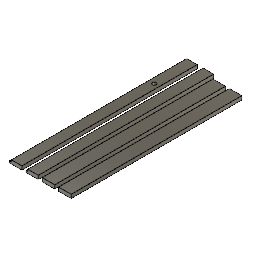
side (Autodesk Fusion 360 design; units mm, degrees)
Autodesk Fusion 360 part; units mm, degrees
sketch "Sketch1" plane through (0, 0, 0) normal (0, 0, 1) x (1, 0, 0)
  line L0 (0, 0) -> (33, 0)
  line L1 (33, 0) -> (33, 460)
  line L2 (33, 460) -> (0, 460)
  line L3 (0, 460) -> (0, 0)
  line L4 (76, 460) -> (43, 460)
  line L5 (43, 460) -> (43, 0)
  line L6 (43, 0) -> (76, 0)
  line L7 (76, 0) -> (76, 460)
  line L8 (86, 0) -> (119, 0)
  line L9 (119, 0) -> (119, 448)
  line L10 (119, 448) -> (86, 448)
  line L11 (86, 448) -> (86, 0)
  line L12 (129, 0) -> (162, 0)
  line L13 (162, 0) -> (162, 448)
  line L14 (162, 448) -> (129, 448)
  line L15 (129, 448) -> (129, 0)
  circle A0 centre (20, 360) radius 5
  line L16 (5, 0) -> (5, 460)
  line L17 (48, 460) -> (48, 0)
  dimension "d1" = 33
  dimension "d2" = 460
  dimension "d3" = 33
  dimension "d4" = 460
  dimension "d5" = 10
  dimension "d6" = 33
  dimension "d8" = 10
  dimension "d9" = 33
  dimension "d10" = 448
  dimension "d11" = 10
  dimension "d14" = 10
  dimension "d15" = 20
  dimension "d16" = 100
  dimension "d19" = 5
  dimension "d20" = 5
  constraint horizontal L0
  constraint vertical L1
  constraint horizontal L2
  constraint vertical L3
  constraint coincident L0.start L3.end
  constraint horizontal L6
  constraint vertical L7
  constraint horizontal L4
  constraint vertical L5
  constraint horizontal L8
  constraint vertical L9
  constraint horizontal L10
  constraint vertical L11
  constraint horizontal L12
  constraint vertical L13
  constraint horizontal L14
  constraint vertical L15
  constraint coincident L0 L16.start
  constraint coincident L2 L16.end
  constraint perpendicular L2 L16
  constraint coincident L4 L17.start
  constraint coincident L6 L17.end
  constraint perpendicular L6 L17
  measures "d1" distance of L0.start L0.end
  measures "d2" distance of L0.start L2.end
  measures "d3" distance of L6.end L5.end
  measures "d4" distance of L4.end L5.end
  measures "d5" distance of L1 L5
  measures "d6" distance of L8.start L8.end
  measures "d8" distance of L7 L11
  measures "d9" distance of L12.start L12.end
  measures "d10" distance of L12.start L14.end
  measures "d11" distance of L9 L15
  measures "d14" diameter of A0
  measures "d15" distance of L3 A0.centre
  measures "d16" distance of L2 A0.centre
  measures "d19" distance of L3 L16
  measures "d20" distance of L5 L17
extrude "Extrude1" add sketch "Sketch1" along normal blind 10 contours L0 L2 L3 L16 | L0 L1 L2 L16 | L4 L6 L7 L17 | L4 L5 L6 L17 | L8 L9 L10 L11 | L12 L13 L14 L15 | A0 makes body 1 at (54, 306.6667, 0) makes body 2 at (11, 306.6667, 0) makes body 3 at (140, 298.6667, 0) makes body 4 at (97, 298.6667, 0)
extrude "Extrude2" cut sketch "Sketch1" along normal blind 10 contours A0 bodies 2
extrude "Extrude3" cut sketch "Sketch1" against normal blind 5 from surface at 10 contours L0 L2 L3 L16 | L4 L5 L6 L17 bodies 1 2
